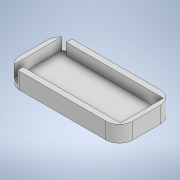
# Autodesk Inventor part: HeadphoneThingy
Saved by Autodesk Inventor 2020 (Build 240168000, 168)
## iProperties
Created: 2020-06-14
Part Number: HeadphoneThingy
Material: Generic
Document SubType Name: Modeling
Designer: Kitte_x
Density: 1 g/cm^3
Appearance: Default
Author: Kitte_x
Autodesk Inventor part; units mm, degrees
ref_plane "YZ Plane" through (0, 0, 0) normal (1, 0, 0) x (0, 1, 0)
ref_plane "XZ Plane" through (0, 0, 0) normal (0, 1, 0) x (-1, 0, 0)
ref_plane "XY Plane" through (0, 0, 0) normal (0, 0, 1) x (1, 0, 0)
sketch "Sketch1" plane through (0, 0, 0) normal (0, 1, 0) x (-1, 0, 0)
  line L0 (10.75, 4.75) -> (-10.75, 4.75) construction
  line L1 (10.75, -4.75) -> (-10.75, -4.75) construction
  line L2 (13.25, 6) -> (13.25, -6)
  line L3 (0, 4.75) -> (0, -4.75) construction
  line L4 (-11.75, 6) -> (-11.75, -6)
  line L5 (-10.75, 4.75) -> (-10.75, -4.75) construction
  line L6 (10.75, 4.75) -> (10.75, -4.75) construction
  line L7 (13.25, 6) -> (-11.75, 6)
  line L8 (13.25, -6) -> (-11.75, -6)
  point P0 (0, 0)
  point P1 (13.25, 0)
  point P2 (0, 0)
  point P3 (0, -4.75)
  point P4 (-11.75, 0)
  dimension "d0" = 9.5
  dimension "d1" = 25
  dimension "d2" = 21.5
  dimension "d3" = 12
  dimension "d4" = 1
  constraints: 18 end point, 6 midpoint, 4 vertical, 3 horizontal, 3 vertical alignment, 2 horizontal alignment, 1 coincident, 1 parallel, 1 perpendicular
  measures "d0" distance between parallel lines of L1 L0
  measures "d1" distance between parallel lines of L4 L2
  measures "d2" distance of L1.start L1.end
  measures "d3" distance of L4.start L4.end
  measures "d4" distance between parallel lines of L4 L5
extrude "Extrusion1" add sketch "Sketch1" against normal blind 1
sketch "Sketch2" plane through (0, 0, 0) normal (0, 1, 0) x (1, 0, 0)
  line L0 (-10.75, 4.75) -> (10.75, 4.75)
  line L1 (-13.25, 6) -> (11.75, 6) projected
  line L2 (10.75, 4.75) -> (10.75, -4.75)
  line L3 (10.75, -4.75) -> (-10.75, -4.75)
  line L4 (-10.75, -4.75) -> (-10.75, -6.052)
  line L5 (-10.75, 4.75) -> (-10.75, 6)
  line L6 (-12.25, -6.052) -> (-12.25, 6)
  line L7 (-13.25, 6) -> (-13.25, -6) projected
  line L8 (-13.25, -6) -> (-13.25, 6) projected
  line L9 (-13.25, -6) -> (-12.25, -6)
  line L10 (-10.75, -6) -> (11.75, -6)
  line L11 (-13.25, 6) -> (-12.25, 6)
  line L12 (-10.75, 6) -> (11.75, 6)
  line L13 (11.75, 6) -> (11.75, -6) projected
  line L14 (11.75, -6) -> (11.75, 6)
  point P0 (0, 0)
  dimension "d7" = 1
  constraints: 22 end point, 4 perpendicular, 4 point on line, 2 collinear, 2 vertical, 1 parallel
  measures "d7" distance between parallel lines of L7 L6
extrude "Extrusion2" add sketch "Sketch2" along normal blind 2.6
fillet "Fillet1" radius 3 2 edges at (11.75, 0.8, 6) (11.75, 0.8, -6)
fillet "Fillet2" radius 3 2 edges at (-13.25, 0.8, -6) (-13.25, 0.8, 6)
body "Solid1"
